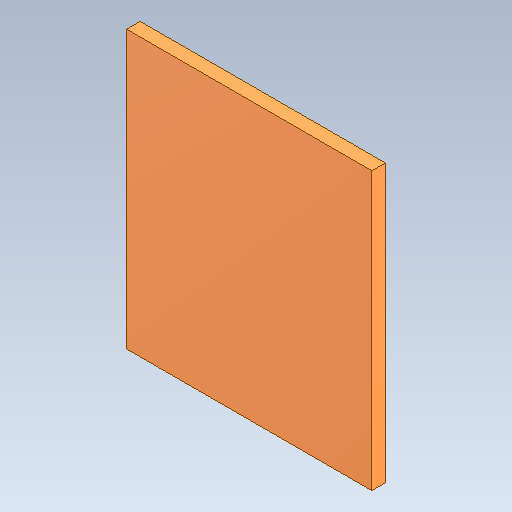
# Autodesk Inventor part: TB6612FNG
Saved by Autodesk Inventor 2020 (Build 240168000, 168)
## iProperties
Created: 2019-07-14
Part Number: TB6612FNG
Material: Generic
Document SubType Name: Modeling
Designer: psrob
Density: 1 g/cm^3
Appearance: TB6612FNG, TB6612FNG
Author: psrob
Autodesk Inventor part; units mm, degrees
ref_plane "YZ Plane" through (0, 0, 0) normal (1, 0, 0) x (0, 1, 0)
ref_plane "XZ Plane" through (0, 0, 0) normal (0, 1, 0) x (-1, 0, 0)
ref_plane "XY Plane" through (0, 0, 0) normal (0, 0, 1) x (1, 0, 0)
sketch "TB6612FNG, TB6612FNG_17" plane through (0, 0, 0) normal (0, 0, 1) x (1, 0, 0)
  line L0 (-8.9535, 7.6835) -> (9.2075, 7.6835)
  line L1 (9.2075, 7.6835) -> (9.2075, -12.827)
  line L2 (9.2075, -12.827) -> (-8.9535, -12.827)
  line L3 (-8.9535, -12.827) -> (-8.9535, 7.6835)
  constraints: 8 end point
extrude "Extrusion1" add sketch "TB6612FNG, TB6612FNG_17" along normal blind 1
body "Solid1"
